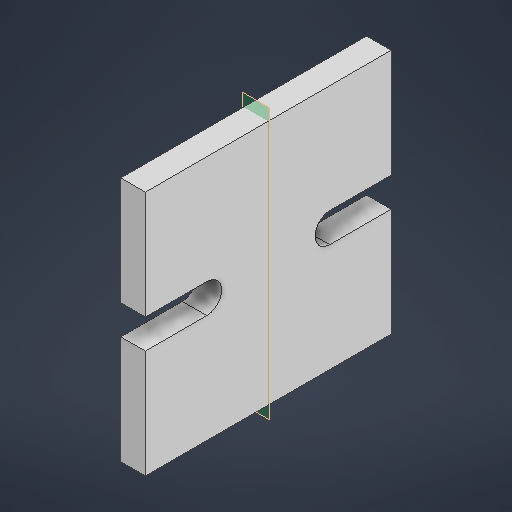
# Autodesk Inventor part: Part3
Saved by Autodesk Inventor 2026 (Build 300175050, 175E)
## iProperties
Created: 2026-04-16
Part Number: Part3
Material: Generic
Document SubType Name: Modeling
Designer: Administrator
Density: 1 g/cm^3
Appearance: Default
Author: Administrator
Autodesk Inventor part; units mm, degrees
ref_plane "YZ Plane" through (0, 0, 0) normal (1, 0, 0) x (0, 1, 0)
ref_plane "XZ Plane" through (0, 0, 0) normal (0, 1, 0) x (-1, 0, 0)
ref_plane "XY Plane" through (0, 0, 0) normal (0, 0, 1) x (1, 0, 0)
sketch "Sketch1" plane through (0, 0, 0) normal (1, 0, 0) x (0, 1, 0)
  line L0 (50, 50) -> (-50, 50)
  line L1 (-50, 50) -> (-50, -50)
  line L2 (-50, -50) -> (50, -50)
  line L3 (50, -50) -> (50, 50)
  line L4 (50, 50) -> (-50, -50) construction
  line L5 (-50, 50) -> (50, -50) construction
  point P0 (0, 0)
  dimension "d0" = 100
  dimension "d1" = 100
  constraints: 12 end point, 2 midpoint, 2 parallel, 1 horizontal, 1 perpendicular
  measures "d0" distance of L0.end L1.end
  measures "d1" distance of L1.end L2.end
extrude "Extrusion1" add sketch "Sketch1" along normal mid plane 10
sketch "Sketch2" plane through (5, 0, 0) normal (1, 0, 0) x (0, 0, -1)
  line L0 (-96.0779, 0) -> (-25, 0) construction
  line L1 (-96.0779, -6) -> (-25, -6)
  line L2 (-25, 6) -> (-96.0779, 6)
  arc A0 (-96.0779, 6) -> (-96.0779, -6) centre (-96.0779, 0) ccw
  arc A1 (-25, -6) -> (-25, 6) centre (-25, 0) ccw
  line L3 (-50, 50) -> (-50, -50) projected
  point P0 (0, 0)
  point P1 (-60.539, 0)
  point P2 (-50, 6)
  point P3 (-50, -6)
  dimension "d4" = 25
  dimension "d5" = 6
  constraints: 8 end point, 4 point on circle, 4 tangent, 2 centre point, 1 horizontal, 1 midpoint, 1 parallel
  measures "d4" distance from line of L0.end L3
  measures "d5" radius of A1
extrude "Extrusion2" cut sketch "Sketch2" along normal through all both and the other way through all contours L3 L2 A1 L1
mirror "Mirror1" about plane through (0, 0, 0) normal (0, 0, 1) of "Extrusion2"
ref_plane "Work Plane1" through (0, 0, 0) normal (0, 0, 1) x (1, 0, 0)
body "Solid1"
